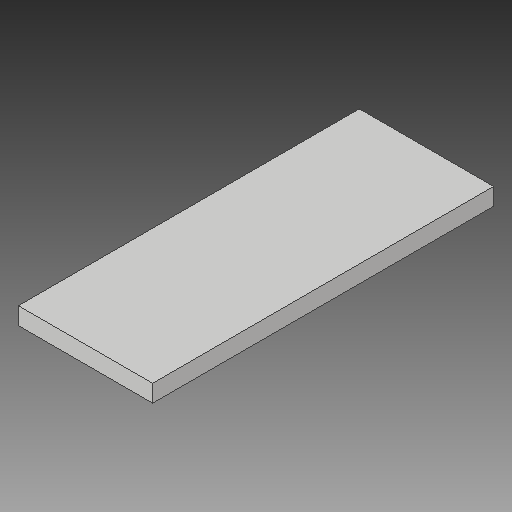
# Autodesk Inventor part: PCB
Saved by Autodesk Inventor 2019 (Build 230136000, 136)
## iProperties
Created: 2022-09-15
Part Number: PCB
Material: Generic
Document SubType Name: Modeling
Designer: ThinkPad
Density: 1 g/cm^3
Appearance: Default
Mass: 19.305 g
Surface Area: 91.02 cm^2
Volume: 19.305 cm^3
Author: ThinkPad
Autodesk Inventor part; units mm, degrees
ref_plane "YZ Plane" through (0, 0, 0) normal (1, 0, 0) x (0, 1, 0)
ref_plane "XZ Plane" through (0, 0, 0) normal (0, 1, 0) x (-1, 0, 0)
ref_plane "XY Plane" through (0, 0, 0) normal (0, 0, 1) x (1, 0, 0)
sketch "Sketch1" plane through (0, 0, 0) normal (0, 1, 0) x (-1, 0, 0)
  line L0 (1.1084, -4.8029) -> (-37.8916, -4.8029)
  line L1 (-37.8916, -4.8029) -> (-37.8916, -103.8029)
  line L2 (-37.8916, -103.8029) -> (1.1084, -103.8029)
  line L3 (1.1084, -103.8029) -> (1.1084, -4.8029)
  point P0 (0, 0)
  dimension "d0" = 39
  dimension "d1" = 99
  constraints: 8 end point, 2 parallel, 1 horizontal, 1 perpendicular
  measures "d0" distance of L2.end L1.end
  measures "d1" distance of L1.end L0.end
extrude "Extrusion1" add sketch "Sketch1" along normal blind 5
body "Solid1"
